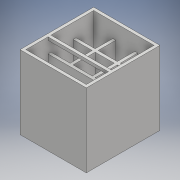
# Autodesk Inventor part: projet
Saved by Autodesk Inventor 2018 (Build 220112000, 112)
## iProperties
Created: 2018-11-20
Part Number: projet
Material: Generic
Document SubType Name: Modeling
Designer: Bienvenue
Density: 1 g/cm^3
Appearance: Default
Author: Bienvenue
Autodesk Inventor part; units mm, degrees
ref_plane "YZ Plane" through (0, 0, 0) normal (1, 0, 0) x (0, 1, 0)
ref_plane "XZ Plane" through (0, 0, 0) normal (0, 1, 0) x (-1, 0, 0)
ref_plane "XY Plane" through (0, 0, 0) normal (0, 0, 1) x (1, 0, 0)
sketch "Sketch1" plane through (0, 0, 0) normal (0, 0, 1) x (1, 0, 0)
  line L0 (0, 0) -> (450, 0)
  line L1 (450, 0) -> (450, 500)
  line L2 (450, 500) -> (0, 500)
  line L3 (0, 500) -> (0, 0)
  dimension "d0" = 500
  dimension "d1" = 450
  constraints: 8 end point, 2 parallel, 1 horizontal, 1 perpendicular
  measures "d0" distance of L0.end L1.end
  measures "d1" distance of L0.start L0.end
extrude "Extrusion1" add sketch "Sketch1" against normal blind 500
sketch "Sketch2" plane through (0, 0, 0) normal (0, 0, 1) x (1, 0, 0)
  line L0 (20, 480) -> (430, 480)
  line L1 (430, 480) -> (430, 20)
  line L2 (430, 20) -> (20, 20)
  line L3 (20, 20) -> (20, 480)
  line L4 (450, 500) -> (0, 500) projected
  line L5 (450, 0) -> (450, 500) projected
  line L6 (0, 500) -> (0, 0) projected
  line L7 (0, 0) -> (450, 0) projected
  dimension "d4" = 20
  dimension "d5" = 20
  dimension "d6" = 20
  dimension "d7" = 20
  constraints: 8 end point, 2 parallel, 1 horizontal, 1 perpendicular
  measures "d4" distance between parallel lines of L4 L0
  measures "d5" distance between parallel lines of L5 L1
  measures "d6" distance between parallel lines of L6 L3
  measures "d7" distance between parallel lines of L7 L2
extrude "Extrusion2" cut sketch "Sketch2" against normal blind 480 contours L0 L1 L2 L3
sketch "Sketch4" plane through (0, 0, 0) normal (0, 0, 1) x (1, 0, 0)
  line L0 (20, 20) -> (20, 480) projected
  line L1 (20, 190) -> (430, 190)
  line L2 (430, 190) -> (430, 170)
  line L3 (430, 170) -> (20, 170)
  line L4 (20, 170) -> (20, 190)
  line L5 (430, 20) -> (20, 20) projected
  point P0 (0, 0)
  dimension "d13" = 410
  dimension "d14" = 20
  dimension "d15" = 150
  constraints: 8 end point, 2 parallel, 1 horizontal, 1 perpendicular, 1 point on line
  measures "d13" distance of L1.start L1.end
  measures "d14" distance of L1.end L2.end
  measures "d15" distance between parallel lines of L5 L3
extrude "Extrusion4" add sketch "Sketch4" against normal blind 20
sketch "Sketch6" plane through (450, 0, 0) normal (1, 0, 0) x (0, 0, -1)
  line L0 (0, 170) -> (20, 170) projected
  line L1 (20, 190) -> (0, 190) projected
  line L2 (20, 170) -> (20, 190) projected
  line L3 (500, 500) -> (500, 0) projected
  line L4 (100, 190) -> (500, 190)
  line L5 (500, 190) -> (500, 170)
  line L6 (500, 170) -> (100, 170)
  line L7 (100, 170) -> (100, 190)
  line L8 (100, 340) -> (500, 340)
  line L9 (500, 340) -> (500, 360)
  line L10 (500, 360) -> (100, 360)
  line L11 (100, 360) -> (100, 340)
  line L12 (0, 0) -> (500, 0) projected
  dimension "d18" = 20
  dimension "d19" = 20
  dimension "d20" = 150
  dimension "d21" = 170
  dimension "d22" = 400
  constraints: 16 end point, 4 parallel, 3 point on line, 2 horizontal, 2 perpendicular
  measures "d18" distance of L10.end L8.start
  measures "d19" distance of L6.end L4.start
  measures "d20" distance between parallel lines of L8 L4
  measures "d21" distance between parallel lines of L12 L6
  measures "d22" distance of L4.start L4.end
extrude "Extrusion6" add sketch "Sketch6" against normal up to surface (430 mm away)
sketch "Sketch7" plane through (0, 0, -480) normal (0, 0, 1) x (1, 0, 0)
  line L0 (430, 360) -> (20, 360) projected
  line L1 (430, 340) -> (20, 340) projected
  line L2 (20, 190) -> (430, 190) projected
  line L3 (430, 170) -> (20, 170) projected
  line L4 (20, 190) -> (430, 190) projected
  line L5 (430, 340) -> (430, 190) projected
  line L6 (430, 340) -> (20, 340) projected
  line L7 (20, 190) -> (20, 340) projected
  line L8 (20, 360) -> (430, 360) projected
  line L9 (430, 480) -> (430, 360) projected
  line L10 (20, 480) -> (430, 480) projected
  line L11 (20, 360) -> (20, 480) projected
  line L12 (430, 170) -> (20, 170) projected
  line L13 (20, 20) -> (20, 170) projected
  line L14 (430, 20) -> (20, 20) projected
  line L15 (430, 170) -> (430, 20) projected
  line L16 (20, 480) -> (430, 480) projected
  line L17 (430, 190) -> (20, 190) projected
  line L18 (150, 480) -> (170, 480)
  line L19 (170, 480) -> (170, 190)
  line L20 (170, 190) -> (150, 190)
  line L21 (150, 190) -> (150, 480)
  line L22 (300, 480) -> (320, 480)
  line L23 (320, 480) -> (320, 190)
  line L24 (320, 190) -> (300, 190)
  line L25 (300, 190) -> (300, 480)
  point P0 (0, 0)
  dimension "d27" = 130
  dimension "d28" = 20
  dimension "d31" = 130
  dimension "d32" = 20
  constraints: 16 end point, 4 parallel, 4 point on line, 2 horizontal, 2 perpendicular
  measures "d27" distance between parallel lines of L11 L21
  measures "d28" distance of L18.start L18.end
  measures "d31" distance between parallel lines of L19 L25
  measures "d32" distance of L22.start L22.end
extrude "Extrusion7" add sketch "Sketch7" along normal up to surface (380 mm away) contours L23 L1 L25 L0 | L0 L25 L10 L23 | L23 L2 L25 L1 | L19 L1 L21 L0 | L0 L21 L10 L19 | L19 L2 L21 L1
body "Solid1"
